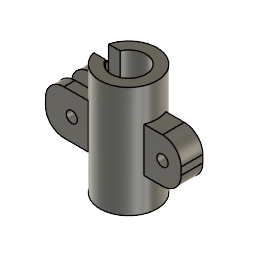
soporte camara (Autodesk Fusion 360 design; units mm, degrees)
Autodesk Fusion 360 part; units mm, degrees
sketch "Boceto1" plane through (0, 0, 64.36) normal (0, 0, 1) x (-1, 0, 0)
  circle A0 centre (-135.6682, 282.303) radius 4.2
  circle A1 centre (-135.6682, 282.303) radius 4.7
  circle A2 centre (-135.6682, 282.303) radius 7.7
  line L0 (-127.9682, 282.303) -> (-143.3682, 282.303) construction
  line L1 (-131.415, 280.303) -> (-128.2325, 280.303)
  line L2 (-131.415, 284.303) -> (-128.2325, 284.303)
  line L3 (-135.6684, 290.003) -> (-135.6684, 274.603) construction
  line L4 (-139.3271, 285.253) -> (-142.7807, 285.253)
  line L5 (-139.3271, 279.353) -> (-142.7807, 279.353)
  line L6 (-142.7807, 285.253) -> (-152.7807, 285.253)
  line L7 (-142.7807, 279.353) -> (-152.7807, 279.353)
  line L8 (-152.7807, 285.253) -> (-152.7807, 279.353)
  dimension "d1" = 0.5
  dimension "d2" = 3
  dimension "d4" = 15.4
  dimension "d5" = 2
  dimension "d6" = 2
  dimension "d15" = 2.95
  dimension "d19" = 10
  constraint coincident A2 L0.start
  constraint coincident A2 L0.end
  constraint horizontal L0
  constraint coincident A1 L1.start
  constraint coincident A2 L1.end
  constraint parallel L0 L1
  constraint coincident A1 L2.start
  constraint coincident A2 L2.end
  constraint horizontal L2
  constraint coincident A2 L3.start
  constraint coincident A2 L3.end
  constraint perpendicular L0 L3
  constraint coincident A1 L4.start
  constraint coincident A2 L4.end
  constraint parallel L0 L4
  constraint symmetric L0 L4.start L5.start
  constraint symmetric L0 L4.end L5.end
  constraint parallel L4 L6
  constraint symmetric L0 L6.end L7.end
  measures "d4" distance of L0.start L0.end
  measures "d5" distance of L0 L1
  measures "d6" distance of L0 L2
  measures "d15" distance of L0 L4
  measures "d19" distance of L4.end L6.end
extrude "Extruir1" add sketch "Boceto1" against normal blind 30 contours A1 A2 L2 L4 | A1 A2 L1 L5 | A1 A2 L4 L5 makes body 1
sketch "Boceto2" plane through (0, 0, 64.36) normal (0, 0, 1) x (-1, 0, 0)
  arc A0 (-131.415, 284.303) -> (-131.415, 280.303) centre (-135.6682, 282.303) ccw
  line L0 (-131.415, 284.303) -> (-128.2325, 284.303)
  arc A1 (-128.2325, 284.303) -> (-128.2325, 280.303) centre (-135.6682, 282.303) ccw
  line L1 (-128.2325, 280.303) -> (-131.415, 280.303)
  circle A2 centre (-135.6682, 282.303) radius 4.2
  line L2 (-128.2325, 284.303) -> (-118.2325, 284.303)
  line L3 (-128.2325, 280.303) -> (-118.2325, 280.303)
  line L4 (-129.8124, 287.303) -> (-118.2325, 287.303)
  line L5 (-135.6682, 282.303) -> (-109, 282.303) construction
  line L6 (-132.4604, 275.303) -> (-118.2325, 275.303)
  line L7 (-118.2325, 287.303) -> (-118.2325, 284.303)
  line L8 (-118.2325, 280.303) -> (-118.2325, 275.303)
  circle A3 centre (-135.6682, 282.303) radius 7.7
  dimension "d9" = 10
  dimension "d10" = 10
  dimension "d11" = 3
  dimension "d34" = 5
  constraint coincident L0.end A1.start
  constraint parallel L0 L2
  constraint coincident A1.end L1.start
  constraint parallel L2 L3
  constraint coincident A1 L4.start
  constraint parallel L2 L4
  constraint coincident A0.centre A1.centre
  constraint horizontal L5
  constraint perpendicular L4 L7
  constraint coincident L6.start A3
  constraint vertical L8
  measures "d9" distance of L0.end L2.end
  measures "d10" distance of A1.end L3.end
  measures "d11" distance of L2 L4
  measures "d34" distance of L3 L6
extrude "Extruir2" add sketch "Boceto2" against normal blind 12 from surface at -9 contours A1 L2 L4 L7 A3 | A1 L3 L6 L8 A3 bodies 1
extrude "Extruir3" add sketch "Boceto1" against normal blind 12 from surface at -9 separate body contours A2 L6 L7 L8 makes body 2
fillet "Empalme1" radius 5 6 edges at (118.2325, -277.803, 55.36) (118.2325, -285.803, 55.36) (118.2325, -277.803, 43.36) (118.2325, -285.803, 43.36) (152.7807, -282.303, 55.36) (152.7807, -282.303, 43.36) on bodies 1 2
sketch "Boceto3" plane through (0, -275.303, 0) normal (0, 1, 0) x (-1, 0, 0)
  arc A0 (-123.2325, 43.36) -> (-118.2325, 48.36) centre (-123.2325, 48.36) ccw
  line L0 (-118.2325, 48.36) -> (-118.2325, 50.36)
  arc A1 (-118.2325, 50.36) -> (-123.2325, 55.36) centre (-123.2325, 50.36) ccw
  line L1 (-123.2325, 55.36) -> (-132.4604, 55.36)
  line L2 (-132.4604, 55.36) -> (-132.4604, 43.36)
  line L3 (-132.4604, 43.36) -> (-123.2325, 43.36)
  arc A2 (-152.7807, 48.36) -> (-147.7807, 43.36) centre (-147.7807, 48.36) ccw
  line L4 (-147.7807, 43.36) -> (-142.7807, 43.36)
  line L5 (-142.7807, 43.36) -> (-142.7807, 55.36)
  line L6 (-142.7807, 55.36) -> (-147.7807, 55.36)
  arc A3 (-147.7807, 55.36) -> (-152.7807, 50.36) centre (-147.7807, 50.36) ccw
  line L7 (-152.7807, 50.36) -> (-152.7807, 48.36)
  line L8 (-125.3464, 55.36) -> (-125.3464, 43.36) construction
  line L9 (-118.2325, 49.36) -> (-132.4604, 49.36) construction
  line L10 (-118.2325, 49.36) -> (-152.7807, 49.36) construction
  line L11 (-135.5066, 76.86) -> (-135.5066, 21.86) construction
  circle A4 centre (-125.3464, 49.36) radius 2
  line L12 (-152.7807, 49.36) -> (-142.7807, 49.36) construction
  line L13 (-122.5464, 50.9766) -> (-125.3464, 52.5932)
  line L14 (-125.3464, 52.5932) -> (-128.1464, 50.9766)
  line L15 (-128.1464, 50.9766) -> (-128.1464, 47.7434)
  line L16 (-128.1464, 47.7434) -> (-125.3464, 46.1268)
  line L17 (-125.3464, 46.1268) -> (-122.5464, 47.7434)
  line L18 (-122.5464, 47.7434) -> (-122.5464, 50.9766)
  circle A5 centre (-147.7807, 49.36) radius 2
  point P0 (-125.3464, 49.36)
  point P1 (-135.5066, 49.36)
  point P2 (-135.5066, 49.36)
  point P3 (-147.7807, 49.36)
  point P4 (-125.3464, 49.36)
  dimension "d22" = 4
  dimension "d23" = 2.8
  dimension "d24" = 4
  constraint midpoint L0 L9.start
  constraint midpoint L2 L9.end
  constraint coincident L1 L8.start
  constraint midpoint L9 P4
  constraint coincident L8 P4
  constraint coincident L3 L8.end
  constraint perpendicular L8 L9
  constraint midpoint L7 L10.end
  constraint vertical L11
  constraint midpoint L10 P2
  constraint coincident L11 P2
  constraint midpoint L11 P2
  constraint coincident P2 P1
  constraint coincident P4 P0
  constraint midpoint L5 L12.end
  constraint midpoint L12 P3
  constraint parallel L0 L15
  constraint coincident P3 A5.centre
  measures "d22" diameter of A4
  measures "d23" distance of P4 L18
  measures "d24" diameter of A5
extrude "Extruir4" cut sketch "Boceto3" against normal up to surface (9.95 mm away) contours A5 bodies 2
extrude "Extruir5" cut sketch "Boceto3" against normal up to surface (2.6 mm away) contours L13 L14 L15 L16 L17 L18 bodies 1
extrude "Extruir6" cut sketch "Boceto3" against normal up to surface (12 mm away) contours A4 bodies 1
sketch "Boceto4" plane through (0, -285.253, 0) normal (0, -1, 0) x (1, 0, 0)
  circle A0 centre (147.7807, 49.36) radius 2
  arc A1 (147.7807, 43.36) -> (152.7807, 48.36) centre (147.7807, 48.36) ccw
  line L0 (152.7807, 48.36) -> (152.7807, 50.36)
  arc A2 (152.7807, 50.36) -> (147.7807, 55.36) centre (147.7807, 50.36) ccw
  line L1 (147.7807, 55.36) -> (142.7807, 55.36)
  line L2 (142.7807, 55.36) -> (142.7807, 43.36)
  line L3 (142.7807, 43.36) -> (147.7807, 43.36)
  circle A3 centre (147.7807, 49.36) radius 1.5
  dimension "d35" = 3
  constraint concentric A0 A3
  measures "d35" diameter of A3
extrude "Extruir7" add sketch "Boceto4" against normal blind 5.9 contours A0 bodies 2
extrude "Extruir8" add 1 faces at (124.0798, -277.903, 47.1661) along direction (0, 1, 0) blind 2.6 on bodies 1 bodies 1
sketch "Boceto5" plane through (0, -275.303, 0) normal (0, 1, 0) x (-1, 0, 0)
  circle A0 centre (-125.3464, 49.36) radius 2
  arc A1 (-123.2325, 43.36) -> (-118.2325, 48.36) centre (-123.2325, 48.36) ccw
  line L0 (-118.2325, 48.36) -> (-118.2325, 50.36)
  arc A2 (-118.2325, 50.36) -> (-123.2325, 55.36) centre (-123.2325, 50.36) ccw
  line L1 (-123.2325, 55.36) -> (-132.4604, 55.36)
  line L2 (-132.4604, 55.36) -> (-132.4604, 43.36)
  line L3 (-132.4604, 43.36) -> (-123.2325, 43.36)
  circle A3 centre (-125.3464, 49.36) radius 1.5
  circle A4 centre (-125.3464, 49.36) radius 2.875
  dimension "d40" = 3
  dimension "d41" = 5.75
  constraint concentric A0 A3
  constraint concentric A3 A4
  measures "d40" diameter of A3
  measures "d41" diameter of A4
extrude "Extruir9" cut sketch "Boceto5" against normal blind 2 contours A4 bodies 1
sketch "Boceto6" plane through (0, -287.303, 0) normal (0, -1, 0) x (1, 0, 0)
  circle A0 centre (125.3464, 49.36) radius 2
  arc A1 (118.2325, 48.36) -> (123.2325, 43.36) centre (123.2325, 48.36) ccw
  line L0 (123.2325, 43.36) -> (129.8124, 43.36)
  line L1 (129.8124, 43.36) -> (129.8124, 55.36)
  line L2 (129.8124, 55.36) -> (123.2325, 55.36)
  arc A2 (123.2325, 55.36) -> (118.2325, 50.36) centre (123.2325, 50.36) ccw
  line L3 (118.2325, 50.36) -> (118.2325, 48.36)
  circle A3 centre (125.3464, 49.36) radius 1.5
  dimension "d44" = 3
  constraint concentric A0 A3
  measures "d44" diameter of A3
extrude "Extruir10" add sketch "Boceto6" against normal blind 3 contours A0 bodies 1
sketch "Boceto7" plane through (0, -280.303, 0) normal (0, -1, 0) x (1, 0, 0)
  circle A0 centre (125.3464, 49.36) radius 2
  arc A1 (118.2325, 48.36) -> (123.2325, 43.36) centre (123.2325, 48.36) ccw
  line L0 (123.2325, 43.36) -> (128.2325, 43.36)
  line L1 (128.2325, 43.36) -> (128.2325, 34.36)
  line L2 (128.2325, 34.36) -> (131.415, 34.36)
  line L3 (131.415, 34.36) -> (131.415, 64.36)
  line L4 (131.415, 64.36) -> (128.2325, 64.36)
  line L5 (128.2325, 64.36) -> (128.2325, 55.36)
  line L6 (128.2325, 55.36) -> (123.2325, 55.36)
  arc A2 (123.2325, 55.36) -> (118.2325, 50.36) centre (123.2325, 50.36) ccw
  line L7 (118.2325, 50.36) -> (118.2325, 48.36)
  circle A3 centre (125.3464, 49.36) radius 1.5
  dimension "d47" = 3
  constraint concentric A0 A3
  measures "d47" diameter of A3
extrude "Extruir11" add sketch "Boceto7" against normal blind 3 contours A0 bodies 1
